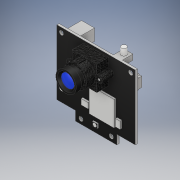
# Autodesk Inventor part: PixyCamKinda
Saved by Autodesk Inventor 2017 (Build 210142000, 142)
## iProperties
Created: 2016-12-06
Part Number: PixyCamKinda
Material: Generic
Document SubType Name: Modeling
Designer: PLTW
Density: 1 g/cm^3
Appearance: Default
Author: PLTW
Autodesk Inventor part; units mm, degrees
ref_plane "YZ Plane" through (0, 0, 0) normal (1, 0, 0) x (0, 1, 0)
ref_plane "XZ Plane" through (0, 0, 0) normal (0, 1, 0) x (-1, 0, 0)
ref_plane "XY Plane" through (0, 0, 0) normal (0, 0, 1) x (1, 0, 0)
sketch "Sketch1" plane through (0, 0, 0) normal (0, 1, 0) x (-1, 0, 0)
  line L0 (-22.225, 26.924) -> (22.225, 26.924)
  line L1 (22.225, 26.924) -> (22.225, -26.924)
  line L2 (22.225, -26.924) -> (-22.225, -26.924)
  line L3 (-22.225, -26.924) -> (-22.225, 26.924)
  line L4 (-22.225, 26.924) -> (22.225, -26.924) construction
  line L5 (22.225, 26.924) -> (-22.225, -26.924) construction
  line L6 (-22.225, 14.224) -> (-28.575, 14.224)
  line L7 (-28.575, 14.224) -> (-28.575, -14.224)
  line L8 (-28.575, -14.224) -> (-22.225, -14.224)
  line L9 (-22.225, -14.224) -> (-22.225, 14.224)
  circle A0 centre (19.05, 23.749) radius 1.524
  circle A1 centre (19.05, -23.749) radius 1.524
  circle A2 centre (-14.097, 23.749) radius 1.524
  circle A3 centre (-25.4, 10.414) radius 1.524
  circle A4 centre (-25.4, -10.414) radius 1.524
  point P0 (0, 0)
  dimension "d0" = 53.848
  dimension "d1" = 44.45
  dimension "d2" = 12.7
  dimension "d3" = 12.7
  dimension "d4" = 6.35
  dimension "d5" = 3.175
  dimension "d6" = 3.175
  dimension "d7" = 3.048
  dimension "d8" = 3.175
  dimension "d9" = 3.048
  dimension "d10" = 8.128
  dimension "d11" = 3.175
  dimension "d12" = 3.81
  dimension "d13" = 3.81
  dimension "d14" = 3.175
  constraints: 20 end point, 5 centre point, 4 parallel, 3 equal radius, 2 horizontal, 2 midpoint, 2 perpendicular, 1 horizontal alignment, 1 point on line, 1 vertical alignment
  measures "d0" distance of L0.end L1.end
  measures "d1" distance of L1.end L2.end
  measures "d2" distance from line of L8 L2.end
  measures "d3" distance from line of L6 L0.start
  measures "d4" distance of L7.end L8.end
  measures "d5" distance from line of L1 A0.centre
  measures "d6" distance from line of A0.centre L0
  measures "d7" diameter of A0
  measures "d8" distance from line of L2 A1.centre
  measures "d9" diameter of A1
  measures "d10" distance from line of L3 A2.centre
  measures "d11" distance from line of L7 A3.centre
  measures "d12" distance from line of L6 A3.centre
  measures "d13" distance from line of L8 A4.centre
  measures "d14" distance from line of L7 A4.centre
extrude "Extrusion1" add sketch "Sketch1" along normal blind 1.524
sketch "Sketch2" plane through (0, 1.524, 0) normal (0, 1, 0) x (1, 0, 0)
  line L0 (-20.6248, 8.509) -> (-3.6068, 8.509)
  line L1 (-3.6068, 8.509) -> (-3.6068, -8.509)
  line L2 (-3.6068, -8.509) -> (-20.6248, -8.509)
  line L3 (-20.6248, -8.509) -> (-20.6248, 8.509)
  line L4 (-12.1158, 10.0203) -> (-12.1158, -10.0203) construction
  arc A0 (-9.8933, 10.0203) -> (-14.3383, 10.0203) centre (-12.1158, 10.0203) ccw
  arc A1 (-14.3383, -10.0203) -> (-9.8933, -10.0203) centre (-12.1158, -10.0203) ccw
  circle A2 centre (-12.1158, 10.0203) radius 0.762
  circle A3 centre (-12.1158, -10.0203) radius 0.762
  line L5 (-14.3383, 10.0203) -> (-14.3383, 8.509)
  line L6 (-14.3383, -8.509) -> (-14.3383, -10.0203)
  line L7 (-9.8933, -10.0203) -> (-9.8933, -8.509)
  line L8 (-9.8933, 8.509) -> (-9.8933, 10.0203)
  line L9 (-22.225, 26.924) -> (-22.225, -26.924) projected
  point P0 (0, 0)
  point P1 (-12.1158, 0)
  dimension "d17" = 17.018
  dimension "d18" = 4.445
  dimension "d19" = 24.4856
  dimension "d20" = 1.6002
  dimension "d21" = 1.524
  dimension "d22" = 8.509
  constraints: 20 end point, 8 tangent, 6 parallel, 4 centre point, 4 point on circle, 4 point on line, 3 vertical alignment, 2 coincident, 2 equal length, 1 equal radius, 1 horizontal, 1 horizontal alignment, 1 midpoint, 1 perpendicular, 1 vertical
  measures "d17" distance of L0.start L0.end
  measures "d18" distance between parallel lines of L8 L5
  measures "d20" distance between parallel lines of L3 L9
  measures "d21" diameter of A2
  measures "d22" distance between parallel lines of L3 L4
extrude "Extrusion2" add sketch "Sketch2" along normal blind 7.9756
sketch "Sketch3" plane through (0, 9.4996, 0) normal (0, 1, 0) x (1, 0, 0)
  circle A0 centre (-12.1158, 0) radius 7.493
  circle A1 centre (-12.1158, -10.0203) radius 0.762 projected
  circle A2 centre (-12.1158, 10.0203) radius 0.762 projected
  line L0 (-14.3383, 10.0203) -> (-14.3383, 8.509) projected
  line L1 (-14.3383, 8.509) -> (-20.6248, 8.509) projected
  line L2 (-20.6248, 8.509) -> (-20.6248, -8.509) projected
  line L3 (-20.6248, -8.509) -> (-14.3383, -8.509) projected
  line L4 (-14.3383, -8.509) -> (-14.3383, -10.0203) projected
  arc A3 (-14.3383, -10.0203) -> (-9.8933, -10.0203) centre (-12.1158, -10.0203) ccw projected
  line L5 (-9.8933, -10.0203) -> (-9.8933, -8.509) projected
  line L6 (-9.8933, -8.509) -> (-3.6068, -8.509) projected
  line L7 (-3.6068, -8.509) -> (-3.6068, 8.509) projected
  line L8 (-3.6068, 8.509) -> (-9.8933, 8.509) projected
  line L9 (-9.8933, 8.509) -> (-9.8933, 10.0203) projected
  arc A4 (-9.8933, 10.0203) -> (-14.3383, 10.0203) centre (-12.1158, 10.0203) ccw projected
  line L10 (-14.6493, 1.4605) -> (-20.6248, 1.4605)
  line L11 (-20.6248, 1.4605) -> (-20.6248, -1.4605)
  line L12 (-20.6248, -1.4605) -> (-14.6493, -1.4605)
  line L13 (-14.6493, -1.4605) -> (-14.6493, 1.4605)
  line L14 (-14.6493, 1.4605) -> (-20.6248, -1.4605) construction
  line L15 (-20.6248, 1.4605) -> (-14.6493, -1.4605) construction
  point P0 (0, 0)
  point P1 (-20.6248, 0)
  point P2 (-17.6371, 0)
  point P3 (-17.6371, 0)
  dimension "d25" = 14.986
  dimension "d26" = 2.921
  constraints: 12 end point, 4 midpoint, 2 horizontal alignment, 2 parallel, 1 centre point, 1 horizontal, 1 perpendicular, 1 point on line, 1 vertical alignment
  measures "d25" diameter of A0
  measures "d26" distance of L10.end L11.end
extrude "Extrusion3" add sketch "Sketch3" along normal blind 6.0452 draft 0.238 contours A0 L12 L13 L10 | L10 L13 L12 A0 | A0 L12 L2 L10
sketch "Sketch4" plane through (0, 15.5448, 0) normal (0, 1, 0) x (1, 0, 0)
  arc A0 (-19.4857, -1.4856) -> (-19.4857, 1.4856) centre (-12.1158, 0) ccw projected
  line L0 (-20.6499, 1.4856) -> (-19.4857, 1.4856) projected
  line L1 (-20.6499, -1.4856) -> (-20.6499, 1.4856) projected
  line L2 (-19.4857, -1.4856) -> (-20.6499, -1.4856) projected
  circle A1 centre (-12.1158, 0) radius 7.0104
  point P0 (0, 0)
  dimension "d29" = 14.0208
  constraints: 1 centre point, 1 coincident
  measures "d29" diameter of A1
extrude "Extrusion4" add sketch "Sketch4" along normal blind 6.5989 contours A1
ref_plane "Work Plane1" through (-12.1158, 15.5448, 0) normal (-1, 0, 0) x (0, 1, 0)
sketch "Sketch5" plane through (-12.1158, 15.5448, 0) normal (-1, 0, 0) x (0, 1, 0)
  line L0 (6.5989, -7.0104) -> (6.5989, 7.0104) projected
  line L1 (0, 7.0104) -> (0, -7.0104) projected
  line L2 (6.5989, -5.8166) -> (5.3543, -4.572)
  line L3 (6.5989, 0) -> (5.5829, 0)
  line L4 (6.5989, -5.8166) -> (6.5989, 0)
  line L5 (6.5989, -7.0104) -> (6.5989, 7.0104) projected
  arc A0 (5.3543, -4.572) -> (6.0909, 0) centre (-8.4663, 0) ccw
  line L6 (-19.9735, 0) -> (11.0277, 0) projected
  point P0 (-15.5448, 0)
  dimension "d33" = 1.1938
  dimension "d34" = 2.4384
  dimension "d35" = 135
  dimension "d36" = 0.508
  constraints: 6 end point, 2 midpoint, 2 point on circle, 1 centre point, 1 collinear, 1 horizontal, 1 horizontal alignment, 1 point on line
  measures "d33" distance of L2.start L0.start
  measures "d34" vertical distance of L0.start L2.end
  measures "d35" angle of L2 L0
  measures "d36" distance of A0.end L3.start
revolve "Revolution1" cut sketch "Sketch5" angle 360 about axis through (-12.1158, 15.5448, 0) along (0, 1, 0)
sketch "Sketch6" plane through (0, 1.524, 0) normal (0, 1, 0) x (1, 0, 0)
  line L0 (21.9431, 1.7526) -> (24.765, 1.7526)
  line L1 (24.765, 1.7526) -> (24.765, -1.7526)
  line L2 (24.765, -1.7526) -> (21.9431, -1.7526)
  line L3 (21.9431, -1.7526) -> (21.9431, 1.7526)
  line L4 (21.9431, 1.7526) -> (24.765, -1.7526) construction
  line L5 (24.765, 1.7526) -> (21.9431, -1.7526) construction
  line L6 (28.575, -14.224) -> (28.575, 14.224) projected
  point P0 (0, 0)
  point P1 (23.354, 0)
  point P2 (23.354, 0)
  dimension "d38" = 2.8219
  dimension "d39" = 3.5052
  dimension "d40" = 3.81
  constraints: 12 end point, 3 midpoint, 2 parallel, 1 horizontal, 1 horizontal alignment, 1 perpendicular
  measures "d38" distance of L0.start L0.end
  measures "d39" distance of L2.end L0.start
  measures "d40" distance between parallel lines of L6 L1
extrude "Extrusion5" add sketch "Sketch6" along normal blind 0.9652
sketch "Sketch7" plane through (0, 2.4892, 0) normal (0, 1, 0) x (1, 0, 0)
  circle A0 centre (23.354, 0) radius 1.3208
  line L0 (21.9431, -1.7526) -> (24.765, -1.7526) projected
  point P0 (0, 0)
  point P1 (23.354, -1.7526)
  dimension "d43" = 2.6416
  constraints: 1 centre point, 1 horizontal alignment, 1 midpoint, 1 vertical alignment
  measures "d43" diameter of A0
extrude "Extrusion6" cut sketch "Sketch7" against normal blind 0.0025
sketch "Sketch8" plane through (0, 0, 0) normal (0, -1, 0) x (1, 0, 0)
  line L0 (-22.225, -16.5862) -> (-18.542, -16.5862)
  line L1 (-18.542, -16.5862) -> (-18.542, -10.3632)
  line L2 (-18.542, -10.3632) -> (-22.225, -10.3632)
  line L3 (-22.225, -10.3632) -> (-22.225, -16.5862)
  line L4 (-22.225, -26.924) -> (-22.225, 26.924) projected
  line L5 (22.225, -26.924) -> (-22.225, -26.924) projected
  point P0 (0, 0)
  dimension "d46" = 6.223
  dimension "d47" = 3.683
  dimension "d48" = 10.3378
  constraints: 8 end point, 2 parallel, 1 horizontal, 1 perpendicular, 1 point on line
  measures "d46" distance of L2.end L0.start
  measures "d47" distance of L0.start L0.end
  measures "d48" distance between parallel lines of L5 L0
extrude "Extrusion7" add sketch "Sketch8" along normal blind 7.2136
sketch "Sketch9" plane through (-22.225, 0, 26.924) normal (-1, 0, 0) x (0, 0, 1)
  circle A0 centre (-40.3987, -4.1021) radius 1.7145
  line L0 (-37.2872, -7.2136) -> (-43.5102, -7.2136) projected
  line L1 (-43.5102, 0) -> (-43.5102, -7.2136) projected
  point P0 (-26.924, 0)
  point P1 (-40.3987, -7.2136)
  dimension "d51" = 3.1115
  dimension "d52" = 3.1115
  dimension "d53" = 3.429
  constraints: 1 centre point, 1 midpoint, 1 vertical alignment
  measures "d51" distance from line of L1 A0.centre
  measures "d52" distance from line of L0 A0.centre
  measures "d53" diameter of A0
extrude "Extrusion8" add sketch "Sketch9" along normal blind 4.3942
sketch "Sketch10" plane through (0, 0, 0) normal (0, -1, 0) x (1, 0, 0)
  line L0 (-10.4152, -20.4482) -> (-2.7952, -20.4482)
  line L1 (-2.7952, -20.4482) -> (-2.7952, -16.435)
  line L2 (-2.7952, -16.435) -> (-10.4152, -16.435)
  line L3 (-10.4152, -16.435) -> (-10.4152, -20.4482)
  point P0 (0, 0)
  dimension "d56" = 4.0132
  dimension "d57" = 7.62
  constraints: 8 end point, 2 parallel, 1 horizontal, 1 perpendicular
  measures "d56" distance of L2.end L0.start
  measures "d57" distance of L0.start L0.end
extrude "Extrusion9" add sketch "Sketch10" along normal blind 9.3726
sketch "Sketch11" plane through (0, -9.3726, 0) normal (0, -1, 0) x (1, 0, 0)
  line L0 (-10.4152, -20.4482) -> (-2.7952, -20.4482) projected
  line L1 (-2.7952, -20.4482) -> (-2.7952, -16.435) projected
  line L2 (-2.7952, -16.435) -> (-10.4152, -16.435) projected
  line L3 (-10.4152, -16.435) -> (-10.4152, -20.4482) projected
  line L4 (-6.6052, -20.4482) -> (-6.6052, -16.435) construction
  line L5 (-10.4152, -16.435) -> (-2.7952, -16.435) construction
  line L6 (-9.958, -20.4482) -> (-9.958, -19.0682)
  line L7 (-9.958, -19.0682) -> (-10.4152, -18.4416)
  line L8 (-9.958, -20.4482) -> (-10.4152, -20.4482)
  line L9 (-10.4152, -20.4482) -> (-2.7952, -20.4482) projected
  line L10 (-10.4152, -20.4482) -> (-10.4152, -18.4416)
  line L11 (-10.4152, -16.435) -> (-10.4152, -20.4482) projected
  line L12 (-3.2524, -20.4482) -> (-3.2524, -19.0682)
  line L13 (-3.2524, -19.0682) -> (-2.7952, -18.4416)
  line L14 (-3.2524, -20.4482) -> (-2.7952, -20.4482)
  line L15 (-2.7952, -20.4482) -> (-2.7952, -18.4416)
  point P0 (0, 0)
  dimension "d60" = 0.4572
  dimension "d61" = 1.38
  constraints: 18 end point, 5 midpoint, 4 symmetric about line, 2 vertical, 1 horizontal, 1 point on line
  measures "d60" distance between parallel lines of L3 L6
  measures "d61" distance of L6.start L6.end
extrude "Extrusion10" cut sketch "Sketch11" against normal blind 2.54 contours L3 L7 L6 L0
ref_plane "Work Plane2" through (-6.6052, 0, -20.4482) normal (-1, 0, 0) x (0, 0, 1)
mirror "Mirror1" about plane through (-6.6052, 0, -20.4482) normal (-1, 0, 0) of "Extrusion10"
sketch "Sketch12" plane through (0, 0, 0) normal (0, -1, 0) x (1, 0, 0)
  line L0 (-20.9804, 13.3604) -> (-0.6604, 13.3604)
  line L1 (-0.6604, 13.3604) -> (-0.6604, 22.2504)
  line L2 (-0.6604, 22.2504) -> (-20.9804, 22.2504)
  line L3 (-20.9804, 22.2504) -> (-20.9804, 13.3604)
  line L4 (-22.225, 26.924) -> (22.225, 26.924) projected
  line L5 (-22.225, -10.3632) -> (-22.225, 26.924) projected
  point P0 (0, 0)
  dimension "d64" = 8.89
  dimension "d65" = 20.32
  dimension "d66" = 4.6736
  dimension "d67" = 1.2446
  constraints: 8 end point, 2 parallel, 1 horizontal, 1 perpendicular
  measures "d64" distance of L2.end L0.start
  measures "d65" distance of L0.start L0.end
  measures "d66" distance between parallel lines of L2 L4
  measures "d67" distance between parallel lines of L5 L3
extrude "Extrusion11" add sketch "Sketch12" along normal blind 10.7696
sketch "Sketch13" plane through (0, -10.7696, 0) normal (0, -1, 0) x (1, 0, 0)
  line L0 (-20.9804, 13.3604) -> (-0.6604, 13.3604) projected
  line L1 (-0.6604, 13.3604) -> (-0.6604, 22.2504) projected
  line L2 (-0.6604, 22.2504) -> (-20.9804, 22.2504) projected
  line L3 (-20.9804, 22.2504) -> (-20.9804, 13.3604) projected
  line L4 (-19.9644, 14.3764) -> (-1.6764, 14.3764)
  line L5 (-1.6764, 14.3764) -> (-1.6764, 21.2344)
  line L6 (-1.6764, 21.2344) -> (-19.9644, 21.2344)
  line L7 (-19.9644, 21.2344) -> (-19.9644, 14.3764)
  line L8 (-8.6106, 14.3764) -> (-13.0302, 14.3764)
  line L9 (-13.0302, 14.3764) -> (-13.0302, 13.3604)
  line L10 (-13.0302, 13.3604) -> (-8.6106, 13.3604)
  line L11 (-8.6106, 13.3604) -> (-8.6106, 14.3764)
  line L12 (-8.6106, 14.3764) -> (-13.0302, 13.3604) construction
  line L13 (-13.0302, 14.3764) -> (-8.6106, 13.3604) construction
  point P0 (0, 0)
  point P1 (-10.8204, 13.8684)
  point P2 (-10.8204, 13.8684)
  point P3 (-10.8204, 21.2344)
  dimension "d70" = 1.016
  dimension "d71" = 4.4196
  constraints: 20 end point, 4 midpoint, 2 parallel, 2 point on line, 1 horizontal, 1 perpendicular, 1 vertical alignment, 3 other
  measures "d70" distance between parallel lines of L7 L3
  measures "d71" distance between parallel lines of L11 L9
extrude "Extrusion12" cut sketch "Sketch13" against normal blind 6.6294 contours L9 L4 L11 L0 | L4 L7 L6 L5
chamfer "Chamfer1" distance 0.508 angle 45 5 edges at (-19.9644, -10.7696, 17.8054) (-16.4973, -10.7696, 14.3764) (-10.8204, -10.7696, 21.2344) (-1.6764, -10.7696, 17.8054) (-5.1435, -10.7696, 14.3764)
sketch "Sketch14" plane through (0, -4.1402, 0) normal (0, -1, 0) x (1, 0, 0)
  line L0 (-16.5354, 16.8529) -> (-15.9004, 16.8529)
  line L1 (-15.9004, 16.8529) -> (-15.9004, 16.2179)
  line L2 (-15.9004, 16.2179) -> (-16.5354, 16.2179)
  line L3 (-16.5354, 16.2179) -> (-16.5354, 16.8529)
  line L4 (-16.5354, 16.8529) -> (-15.9004, 16.2179) construction
  line L5 (-15.9004, 16.8529) -> (-16.5354, 16.2179) construction
  line L6 (-19.9644, 14.3764) -> (-19.9644, 21.2344) construction
  line L7 (-19.9644, 17.8054) -> (-1.6637, 17.8054) construction
  line L8 (-19.9644, 21.2344) -> (-1.6764, 21.2344) construction
  line L9 (-10.8204, 21.2344) -> (-10.8204, 13.4329) construction
  point P0 (0, 0)
  point P1 (-16.2179, 16.5354)
  dimension "d77" = 0.635
  dimension "d78" = 1.27
  dimension "d79" = 5.08
  constraints: 16 end point, 4 midpoint, 2 horizontal, 2 parallel, 2 perpendicular, 1 vertical
  measures "d77" distance of L2.end L0.start
  measures "d78" distance from line of L7 point (-16.218, 16.535)
  measures "d79" distance between parallel lines of L9 L1
extrude "Extrusion13" add sketch "Sketch14" along normal blind 6.096
chamfer "Chamfer2" distance 0.254 angle 45 4 edges at (-15.9004, -10.2362, 16.5354) (-16.2179, -10.2362, 16.8529) (-16.2179, -10.2362, 16.2179) (-16.5354, -10.2362, 16.5354)
pattern_linear "Rectangular Pattern1" count 5 spacing 2.54 along (1, 0, 0) count 2 spacing 2.54 along (0, 0, 1) of "Extrusion13", "Chamfer2"
sketch "Sketch15" plane through (0, -9.3726, 0) normal (0, -1, 0) x (1, 0, 0)
  line L0 (-3.2524, -19.0682) -> (-2.7952, -18.4416) projected
  line L1 (-2.7952, -18.4416) -> (-2.7952, -16.435) projected
  line L2 (-2.7952, -16.435) -> (-10.4152, -16.435) projected
  line L3 (-10.4152, -16.435) -> (-10.4152, -18.4416) projected
  line L4 (-10.4152, -18.4416) -> (-9.958, -19.0682) projected
  line L5 (-9.958, -19.0682) -> (-9.958, -20.4482) projected
  line L6 (-9.958, -20.4482) -> (-3.2524, -20.4482) projected
  line L7 (-3.2524, -20.4482) -> (-3.2524, -19.0682) projected
  line L8 (-10.0342, -18.3174) -> (-10.0342, -16.816)
  line L9 (-10.0342, -16.816) -> (-3.1762, -16.816)
  line L10 (-3.1762, -16.816) -> (-3.1762, -18.3174)
  line L11 (-3.1762, -18.3174) -> (-3.6334, -18.944)
  line L12 (-3.6334, -18.944) -> (-3.6334, -20.0672)
  line L13 (-3.6334, -20.0672) -> (-9.577, -20.0672)
  line L14 (-9.577, -20.0672) -> (-9.577, -18.944)
  line L15 (-9.577, -18.944) -> (-10.0342, -18.3174)
  point P0 (0, 0)
  dimension "d91" = 0.381
  constraints: 16 end point, 7 other
  measures "d91" distance between parallel lines of L3 L8
extrude "Extrusion14" cut sketch "Sketch15" against normal blind 6.096 contours L8 L9 L10 L11 L12 L13 L14 L15
sketch "Sketch16" plane through (0, 0, 0) normal (0, -1, 0) x (1, 0, 0)
  line L0 (7.5438, 12.9032) -> (9.9568, 12.9032)
  line L1 (9.9568, 12.9032) -> (9.9568, 17.8054)
  line L2 (9.9568, 17.8054) -> (7.5438, 17.8054)
  line L3 (7.5438, 17.8054) -> (7.5438, 12.9032)
  line L4 (-22.225, 26.924) -> (22.225, 26.924) projected
  line L5 (-0.6604, 13.3604) -> (-0.6604, 22.2504) projected
  point P0 (0, 0)
  dimension "d94" = 2.413
  dimension "d95" = 4.9022
  dimension "d96" = 9.1186
  dimension "d97" = 8.2042
  constraints: 8 end point, 2 parallel, 1 horizontal, 1 perpendicular
  measures "d94" distance of L0.start L0.end
  measures "d95" distance of L2.end L0.start
  measures "d96" distance between parallel lines of L4 L2
  measures "d97" distance between parallel lines of L3 L5
extrude "Extrusion15" add sketch "Sketch16" along normal blind 3.7338
fillet "Fillet1" radius 0.762 4 edges at (7.5438, -1.8669, 12.9032) (9.9568, -1.8669, 12.9032) (7.5438, -1.8669, 17.8054) (9.9568, -1.8669, 17.8054)
sketch "Sketch17" plane through (0, -3.7338, 0) normal (0, -1, 0) x (1, 0, 0)
  arc A0 (9.9568, 17.0434) -> (9.1948, 17.8054) centre (9.1948, 17.0434) ccw projected
  line L0 (9.1948, 17.8054) -> (8.3058, 17.8054) projected
  arc A1 (8.3058, 17.8054) -> (7.5438, 17.0434) centre (8.3058, 17.0434) ccw projected
  line L1 (7.5438, 17.0434) -> (7.5438, 13.6652) projected
  arc A2 (7.5438, 13.6652) -> (8.3058, 12.9032) centre (8.3058, 13.6652) ccw projected
  line L2 (8.3058, 12.9032) -> (9.1948, 12.9032) projected
  arc A3 (9.1948, 12.9032) -> (9.9568, 13.6652) centre (9.1948, 13.6652) ccw projected
  line L3 (9.9568, 13.6652) -> (9.9568, 17.0434) projected
  line L4 (8.4328, 13.7668) -> (9.0678, 13.7668)
  line L5 (9.0678, 13.7668) -> (9.0678, 14.4018)
  line L6 (9.0678, 14.4018) -> (8.4328, 14.4018)
  line L7 (8.4328, 14.4018) -> (8.4328, 13.7668)
  line L8 (8.4328, 13.7668) -> (9.0678, 14.4018) construction
  line L9 (9.0678, 13.7668) -> (8.4328, 14.4018) construction
  line L10 (7.5438, 17.0434) -> (7.5438, 13.6652) construction
  line L11 (7.5438, 15.3543) -> (9.9568, 15.3543) construction
  point P0 (0, 0)
  point P1 (8.7503, 14.0843)
  point P2 (8.7503, 12.9032)
  point P3 (8.7503, 14.0843)
  dimension "d104" = 1.27
  dimension "d105" = 0.635
  constraints: 14 end point, 7 midpoint, 2 horizontal, 2 parallel, 2 perpendicular, 1 vertical alignment
  measures "d104" distance from line of L11 point (8.75, 14.084)
  measures "d105" distance of L4.start L4.end
extrude "Extrusion16" add sketch "Sketch17" along normal blind 5.9182 contours L7 L6 L5 L4
chamfer "Chamfer3" distance 0.254 angle 45 4 edges at (8.7503, -9.652, 13.7668) (8.4328, -9.652, 14.0843) (8.7503, -9.652, 14.4018) (9.0678, -9.652, 14.0843)
pattern_linear "Rectangular Pattern3" count 2 spacing 2.54 along (0, 0, 1) of "Extrusion16", "Chamfer3"
pattern_linear "Rectangular Pattern4" count 3 spacing 2.4155 along (1, 0, 0) of "Chamfer3", "Extrusion16", "Rectangular Pattern3", "Extrusion15", "Fillet1"
sketch "Sketch18" plane through (0, 0, 0) normal (0, -1, 0) x (1, 0, 0)
  line L0 (16.0833, 17.8943) -> (21.1633, 17.8943)
  line L1 (21.1633, 17.8943) -> (21.1633, 12.8143)
  line L2 (21.1633, 12.8143) -> (16.0833, 12.8143)
  line L3 (16.0833, 12.8143) -> (16.0833, 17.8943)
  line L4 (16.0833, 17.8943) -> (21.1633, 12.8143) construction
  line L5 (21.1633, 17.8943) -> (16.0833, 12.8143) construction
  line L6 (14.7879, 13.6652) -> (14.7879, 17.0434) projected
  point P0 (0, 0)
  point P1 (18.6233, 15.3543)
  point P2 (18.6233, 15.3543)
  point P3 (14.7879, 15.3543)
  dimension "d117" = 5.08
  dimension "d118" = 1.2954
  constraints: 12 end point, 4 midpoint, 2 parallel, 2 perpendicular, 1 horizontal, 1 horizontal alignment
  measures "d117" distance of L0.end L1.end
  measures "d118" distance between parallel lines of L6 L3
extrude "Extrusion17" add sketch "Sketch18" along normal blind 1.8288
sketch "Sketch19" plane through (0, -1.8288, 0) normal (0, -1, 0) x (1, 0, 0)
  line L0 (18.9408, 16.9418) -> (18.3058, 16.9418)
  line L1 (18.3058, 16.9418) -> (18.3058, 16.3068)
  line L2 (18.3058, 16.3068) -> (18.9408, 16.3068)
  line L3 (18.9408, 16.3068) -> (18.9408, 16.9418)
  line L4 (18.9408, 16.9418) -> (18.3058, 16.3068) construction
  line L5 (18.3058, 16.9418) -> (18.9408, 16.3068) construction
  line L6 (16.0833, 15.3543) -> (21.1633, 15.3543) construction
  line L7 (21.1633, 12.8143) -> (21.1633, 17.8943) construction
  line L8 (16.0833, 17.8943) -> (16.0833, 12.8143) construction
  line L9 (16.0833, 12.8143) -> (21.1633, 12.8143) construction
  point P0 (0, 0)
  point P1 (18.6233, 16.6243)
  point P2 (18.6233, 12.8143)
  point P3 (18.6233, 16.6243)
  dimension "d121" = 1.27
  dimension "d122" = 0.635
  constraints: 14 end point, 6 midpoint, 2 horizontal, 2 parallel, 2 perpendicular, 1 vertical alignment
  measures "d121" distance from line of L6 point (18.623, 16.624)
  measures "d122" distance of L0.end L1.end
extrude "Extrusion18" add sketch "Sketch19" along normal blind 7.4422
chamfer "Chamfer4" distance 0.254 angle 45 4 edges at (18.3058, -9.271, 16.6243) (18.6233, -9.271, 16.3068) (18.9408, -9.271, 16.6243) (18.6233, -9.271, 16.9418)
pattern_linear "Rectangular Pattern5" count 2 spacing 2.54 along (0, 0, -1) of "Extrusion18", "Chamfer4"
sketch "Sketch20" plane through (21.1633, 0, 17.8943) normal (1, 0, 0) x (0, 0, -1)
  line L0 (-0.0635, 0) -> (5.1435, 0)
  line L1 (5.1435, 0) -> (5.1435, -2.3114)
  line L2 (5.1435, -2.3114) -> (-0.0635, -2.3114)
  line L3 (-0.0635, -2.3114) -> (-0.0635, 0)
  line L4 (-0.0635, 0) -> (5.1435, -2.3114) construction
  line L5 (5.1435, 0) -> (-0.0635, -2.3114) construction
  line L6 (3.6703, 0) -> (32.1183, 0) projected
  line L7 (0, -1.8288) -> (5.08, -1.8288) projected
  line L8 (1.2065, -7.3914) -> (3.8735, -7.3914)
  line L9 (3.8735, -7.3914) -> (3.8735, -2.3114)
  line L10 (3.8735, -2.3114) -> (1.2065, -2.3114)
  line L11 (1.2065, -2.3114) -> (1.2065, -7.3914)
  line L12 (1.2065, -7.3914) -> (3.8735, -2.3114) construction
  line L13 (3.8735, -7.3914) -> (1.2065, -2.3114) construction
  point P0 (17.8943, 0)
  point P1 (2.54, -1.1557)
  point P2 (2.54, -1.1557)
  point P3 (2.54, -1.8288)
  point P4 (2.54, -4.8514)
  point P5 (2.54, -4.8514)
  point P6 (2.54, -1.1557)
  dimension "d131" = 5.207
  dimension "d132" = 2.3114
  dimension "d133" = 2.667
  dimension "d134" = 5.08
  constraints: 24 end point, 8 midpoint, 4 parallel, 2 horizontal, 2 perpendicular, 2 point on line, 2 vertical alignment
  measures "d131" distance of L1.end L2.end
  measures "d132" distance of L0.end L1.end
  measures "d133" distance of L8.start L8.end
  measures "d134" distance between parallel lines of L10 L8
extrude "Extrusion19" add sketch "Sketch20" along normal blind 0.9144
sketch "Sketch21" plane through (21.1633, -7.3914, 14.0208) normal (0, 0, -1) x (-1, 0, 0)
  line L0 (0, 3.429) -> (1.0668, 1.7145)
  line L1 (1.0668, 1.7145) -> (0, 0)
  line L2 (0, 0) -> (0, 5.08) projected
  line L3 (-0.9144, 0) -> (-0.9144, 5.08) projected
  point P0 (21.1633, 7.3914)
  dimension "d137" = 3.429
  dimension "d138" = 1.9812
  constraints: 4 end point, 1 equal length, 1 point on line
  measures "d137" distance of L1.end L0.start
  measures "d138" distance from line of L3 L0.end
extrude "Extrusion20" add sketch "Sketch21" against normal up to surface (2.667 mm away)
fillet "Fillet2" radius 0.762 4 edges at (21.1633, -7.3914, 15.3543) (22.0777, -7.3914, 15.3543) (20.0965, -5.6769, 15.3543) (21.1633, -3.9624, 15.3543)
sketch "Sketch22" plane through (0, 1.524, 0) normal (0, 1, 0) x (1, 0, 0)
  line L0 (1.2192, -3.429) -> (18.2372, -3.429)
  line L1 (18.2372, -3.429) -> (18.2372, 13.589)
  line L2 (18.2372, 13.589) -> (1.2192, 13.589)
  line L3 (1.2192, 13.589) -> (1.2192, -3.429)
  line L4 (11.9888, -9.0424) -> (15.7988, -9.0424)
  line L5 (15.7988, -9.0424) -> (15.7988, -4.2164)
  line L6 (15.7988, -4.2164) -> (11.9888, -4.2164)
  line L7 (11.9888, -4.2164) -> (11.9888, -9.0424)
  line L8 (-3.6068, -8.509) -> (-3.6068, 8.509) projected
  line L9 (22.225, 26.924) -> (-22.225, 26.924) projected
  line L10 (12.065, 14.5034) -> (17.0434, 14.5034)
  line L11 (17.0434, 14.5034) -> (17.0434, 17.7038)
  line L12 (17.0434, 17.7038) -> (12.065, 17.7038)
  line L13 (12.065, 17.7038) -> (12.065, 14.5034)
  line L14 (22.225, 14.224) -> (22.225, 26.924) projected
  line L15 (-22.225, -26.924) -> (22.225, -26.924) projected
  line L16 (28.575, -14.224) -> (28.575, 14.224) projected
  point P0 (0, 0)
  dimension "d142" = 17.018
  dimension "d143" = 4.826
  dimension "d144" = 13.335
  dimension "d145" = 4.9784
  dimension "d146" = 9.2202
  dimension "d147" = 3.2004
  dimension "d148" = 5.1816
  dimension "d149" = 3.81
  dimension "d150" = 4.826
  dimension "d151" = 17.8816
  dimension "d152" = 12.7762
  constraints: 24 end point, 6 parallel, 4 perpendicular, 3 horizontal
  measures "d142" distance of L1.end L2.end
  measures "d143" distance between parallel lines of L8 L3
  measures "d144" distance between parallel lines of L9 L2
  measures "d145" distance of L11.end L12.end
  measures "d146" distance between parallel lines of L9 L12
  measures "d147" distance of L12.end L10.start
  measures "d148" distance between parallel lines of L14 L11
  measures "d149" distance between parallel lines of L5 L7
  measures "d150" distance of L6.end L4.start
  measures "d151" distance between parallel lines of L4 L15
  measures "d152" distance between parallel lines of L16 L5
extrude "Extrusion21" add sketch "Sketch22" along normal blind 1.27
sketch "Sketch23" plane through (0, 1.524, 0) normal (0, 1, 0) x (1, 0, 0)
  line L0 (5.8674, -20.4724) -> (11.8364, -20.4724)
  line L1 (11.8364, -20.4724) -> (11.8364, -14.097)
  line L2 (11.8364, -14.097) -> (5.8674, -14.097)
  line L3 (5.8674, -14.097) -> (5.8674, -20.4724)
  line L4 (-22.225, -26.924) -> (22.225, -26.924) projected
  line L5 (22.225, -26.924) -> (22.225, -14.224) projected
  point P0 (0, 0)
  dimension "d155" = 5.969
  dimension "d156" = 6.3754
  dimension "d157" = 6.4516
  dimension "d158" = 10.3886
  constraints: 8 end point, 2 parallel, 1 horizontal, 1 perpendicular
  measures "d155" distance of L0.start L0.end
  measures "d156" distance of L2.end L0.start
  measures "d157" distance between parallel lines of L4 L0
  measures "d158" distance between parallel lines of L5 L1
extrude "Extrusion22" add sketch "Sketch23" along normal blind 2.3114
sketch "Sketch24" plane through (-12.1158, 15.5448, 0) normal (-1, 0, 0) x (0, 1, 0)
  line L0 (0, -7.0104) -> (6.5989, -7.0104) projected
  line L1 (0, 7.0104) -> (6.5989, 7.0104) projected
  line L2 (0, -7.0104) -> (2.9972, -7.0104)
  line L3 (2.9972, -7.0104) -> (2.9972, -5.9436)
  line L4 (2.9972, -5.9436) -> (0, -5.9436)
  line L5 (0, -5.9436) -> (0, -7.0104)
  line L6 (-19.9735, 0) -> (11.0277, 0) projected
  point P0 (-15.5448, 0)
  dimension "d161" = 2.9972
  dimension "d162" = 5.9436
  constraints: 8 end point, 2 parallel, 1 horizontal, 1 perpendicular
  measures "d161" distance of L3.end L4.end
  measures "d162" distance from line of point (-15.545, 0) L4
revolve "Revolution2" cut sketch "Sketch24" angle 360 about axis through (-12.1158, 15.5448, 0) along (0, 1, 0)
equation "\"d22\" = 0.5 * d17"
equation "\"d52\" = d51"
body "Solid1"
